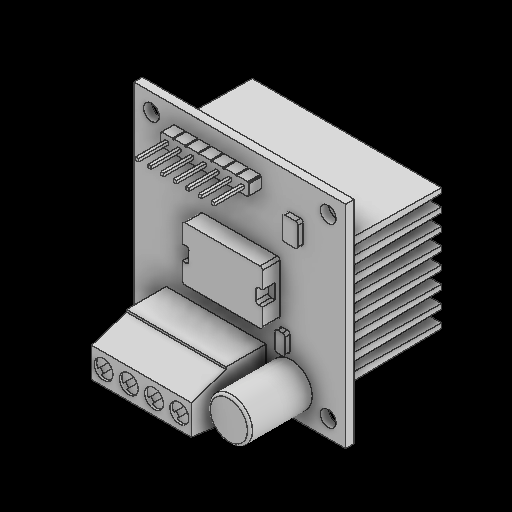
# Autodesk Inventor part: IBTMiniOriginal
Saved by Autodesk Inventor 2025.2 (Build 292293000, 293)
## iProperties
Created: 2023-12-09
Part Number: IBTMiniOriginal
Material: Generic
Document SubType Name: Modeling
Designer: valer
Density: 1 g/cm^3
Appearance: Default
Author: valer
Autodesk Inventor part; units mm, degrees
ref_plane "YZ Plane" through (0, 0, 0) normal (1, 0, 0) x (0, 1, 0)
ref_plane "XZ Plane" through (0, 0, 0) normal (0, 1, 0) x (-1, 0, 0)
ref_plane "XY Plane" through (0, 0, 0) normal (0, 0, 1) x (1, 0, 0)
sketch "Sketch1" plane through (0, 0, 0) normal (0, 0, 1) x (1, 0, 0)
  line L0 (-21.25, 21.25) -> (21.25, 21.25)
  line L1 (21.25, 21.25) -> (21.25, -21.25)
  line L2 (21.25, -21.25) -> (-21.25, -21.25)
  line L3 (-21.25, -21.25) -> (-21.25, 21.25)
  line L4 (-29.75, 0) -> (29.75, 0) construction
  line L5 (0, -29.75) -> (0, 29.75) construction
  point P0 (0, 0)
  point P1 (0, 21.25)
  point P2 (-21.25, 0)
  dimension "d0" = 42.5
  constraints: 8 end point, 2 midpoint, 2 parallel, 2 perpendicular, 2 point on line, 1 horizontal
  measures "d0" distance of L0.start L0.end
extrude "Extrusion1" add sketch "Sketch1" along normal blind 1.7
sketch "Sketch2" plane through (0, 0, 1.7) normal (0, 0, 1) x (1, 0, 0)
  circle A0 centre (-17.75, 17.75) radius 3.5 construction
  line L0 (21.25, 21.25) -> (-21.25, 21.25) construction
  line L1 (-21.25, 21.25) -> (-21.25, -21.25) construction
  circle A1 centre (-17.75, 17.75) radius 1.6
  line L2 (-17.75, 19.35) -> (-17.75, 21.25) construction
  line L3 (-19.35, 17.75) -> (-21.25, 17.75) construction
  line L4 (-29.75, 0) -> (29.75, 0) construction
  line L5 (0, -29.75) -> (0, 29.75) construction
  circle A2 centre (17.75, 17.75) radius 1.6
  circle A3 centre (-17.75, -17.75) radius 1.6
  circle A4 centre (17.75, -17.75) radius 1.6
  point P0 (0, 0)
  dimension "d3" = 1.9
  dimension "d4" = 3.2
  constraints: 5 centre point, 4 end point, 4 point on circle, 3 perpendicular, 3 symmetric about line, 2 point on line, 2 tangent, 1 coincident, 3 other
  measures "d3" distance of L2.start L2.end
  measures "d4" diameter of A1
extrude "Extrusion2" cut sketch "Sketch2" against normal blind 1.7
sketch "Sketch3" plane through (0, 0, 1.7) normal (0, 0, 1) x (1, 0, 0)
  line L0 (-21.25, 21.25) -> (-21.25, -21.25) construction
  line L1 (-21.25, 0) -> (21.25, 0) construction
  line L2 (21.25, -21.25) -> (21.25, 21.25) construction
  line L3 (-8.05, 5.4) -> (8.05, 5.4)
  line L4 (8.05, 5.4) -> (8.05, -5.4)
  line L5 (8.05, -5.4) -> (-8.05, -5.4)
  line L6 (-8.05, -5.4) -> (-8.05, 5.4)
  line L7 (0, -29.75) -> (0, 29.75) construction
  point P0 (0, 0)
  point P1 (-8.05, 0)
  point P2 (0, 5.4)
  dimension "d7" = 16.1
  dimension "d8" = 10.8
  constraints: 10 end point, 4 midpoint, 2 parallel, 2 point on line, 1 horizontal, 1 perpendicular
  measures "d7" distance of L3.start L3.end
  measures "d8" distance of L3.end L4.end
extrude "Extrusion3" add sketch "Sketch3" along normal blind 3.5
sketch "Sketch4" plane through (0, 0, 5.2) normal (0, 0, 1) x (1, 0, 0)
  line L0 (-8.05, -5.4) -> (8.05, -5.4) projected
  line L1 (8.05, -5.4) -> (8.05, 5.4) projected
  line L2 (8.05, 5.4) -> (-8.05, 5.4) projected
  line L3 (-8.05, 5.4) -> (-8.05, -5.4) projected
  line L4 (6.75, 1.5) -> (8.05, 1.5)
  line L5 (8.05, 1.5) -> (8.05, -1.5)
  line L6 (8.05, -1.5) -> (6.75, -1.5)
  line L7 (6.75, -1.5) -> (6.75, 1.5)
  line L8 (0, -29.75) -> (0, 29.75) construction
  line L9 (-6.75, 1.5) -> (-8.05, 1.5)
  line L10 (-8.05, 1.5) -> (-8.05, -1.5)
  line L11 (-8.05, -1.5) -> (-6.75, -1.5)
  line L12 (-6.75, -1.5) -> (-6.75, 1.5)
  point P0 (0, 0)
  point P1 (8.05, 0)
  dimension "d11" = 3
  dimension "d12" = 1.3
  constraints: 16 end point, 4 symmetric about line, 2 midpoint, 2 parallel, 1 horizontal, 1 perpendicular
  measures "d11" distance of L6.end L4.start
  measures "d12" distance of L5.end L6.end
extrude "Extrusion4" cut sketch "Sketch4" against normal blind 2.5 contours L3 L9 L12 L11 | L6 L7 L4 L1
fillet "Fillet1" radius 0.5 4 edges at (6.75, 1.5, 3.95) (6.75, -1.5, 3.95) (-6.75, 1.5, 3.95) (-6.75, -1.5, 3.95)
sketch "Sketch5" plane through (0, 0, 1.7) normal (0, 0, 1) x (1, 0, 0)
  circle A0 centre (10.3, -15.5) radius 4.25
  line L0 (-15.45, -11.25) -> (4.35, -11.25)
  line L1 (4.35, -11.25) -> (4.35, -19.75)
  line L2 (4.35, -19.75) -> (-15.45, -19.75)
  line L3 (-15.45, -19.75) -> (-15.45, -11.25)
  line L4 (-13.45, 17.85) -> (4.35, 17.85)
  line L5 (4.35, 17.85) -> (4.35, 15.25)
  line L6 (4.35, 15.25) -> (-13.45, 15.25)
  line L7 (-13.45, 15.25) -> (-13.45, 17.85)
  line L8 (21.25, 21.25) -> (-21.25, 21.25) projected
  line L9 (-21.25, 21.25) -> (-21.25, -21.25) projected
  line L10 (-15.45, -15.5) -> (14.55, -15.5) construction
  line L11 (4.35, -11.25) -> (10.3, -11.25) construction
  line L12 (-21.25, -21.25) -> (21.25, -21.25) construction
  line L13 (21.25, -21.25) -> (21.25, 21.25) projected
  point P0 (0, 0)
  point P1 (-13.45, 16.55)
  dimension "d16" = 17.8
  dimension "d17" = 2.6
  dimension "d18" = 7.8
  dimension "d19" = 3.4
  dimension "d20" = 30
  dimension "d21" = 8.5
  dimension "d22" = 1.5
  dimension "d23" = 6.7
  constraints: 20 end point, 5 parallel, 2 horizontal, 2 midpoint, 2 perpendicular, 2 point on circle, 2 point on line, 1 centre point, 1 collinear, 1 tangent
  measures "d16" distance of L5.end L6.end
  measures "d17" distance of L4.end L5.end
  measures "d18" distance from line of L9 point (-13.45, 16.55)
  measures "d19" distance between parallel lines of L8 L4
  measures "d20" distance of L10.end L10.start
  measures "d21" distance of L2.end L0.start
  measures "d22" distance between parallel lines of L12 L2
  measures "d23" distance from line of L13 L10.end
extrude "Extrusion5" add sketch "Sketch5" along normal blind 12.5 contours A0
extrude "Extrusion6" add sketch "Sketch5" along normal blind 2.5 contours L4 L5 L6 L7
fillet "Fillet2" radius 0.5 1 edges at (6.05, -15.5, 14.2)
sketch "Sketch8" plane through (0, 0, 1.7) normal (0, 0, 1) x (1, 0, 0)
  line L0 (9.525, 9.525) -> (12.7, 9.525)
  line L1 (12.7, 9.525) -> (12.7, 14.2875)
  line L2 (12.7, 14.2875) -> (9.525, 14.2875)
  line L3 (9.525, 14.2875) -> (9.525, 9.525)
  point P0 (0, 0)
  dimension "d60" = 3.175
  dimension "d61" = 4.7625
  dimension "d62" = 12.7
  dimension "d63" = 14.2875
  constraints: 8 end point, 2 parallel, 1 horizontal, 1 perpendicular
  measures "d60" distance between parallel lines of L1 L3
  measures "d61" distance between parallel lines of L0 L2
  measures "d62" distance from line of point (0, 0) L1
  measures "d63" distance from line of point (0, 0) L2
extrude "Extrusion9" add sketch "Sketch8" along normal blind 1
sketch "Sketch9" plane through (0, 0, 0) normal (0, 0, -1) x (-1, 0, 0)
  line L0 (19, -12.55) -> (-19, -12.55)
  line L1 (-19, -12.55) -> (-19, 12.55)
  line L2 (-19, 12.55) -> (19, 12.55)
  line L3 (19, 12.55) -> (19, -12.55)
  line L4 (29.75, 0) -> (-29.75, 0) projected
  line L5 (0, -29.75) -> (0, 29.75) projected
  point P0 (0, 0)
  point P1 (0, -12.55)
  point P2 (19, 0)
  dimension "d66" = 25.1
  dimension "d67" = 38
  constraints: 8 end point, 2 midpoint, 2 parallel, 2 point on line, 1 horizontal, 1 perpendicular
  measures "d66" distance of L0.end L1.end
  measures "d67" distance of L0.start L0.end
extrude "Extrusion10" add sketch "Sketch9" along normal blind 19.8
sketch "Sketch11" plane through (0, 0, 1.7) normal (0, 0, 1) x (1, 0, 0)
  line L0 (8.05, -6.48) -> (10.05, -6.48)
  line L1 (10.05, -6.48) -> (10.05, -10.48)
  line L2 (10.05, -10.48) -> (8.05, -10.48)
  line L3 (8.05, -10.48) -> (8.05, -6.48)
  line L4 (21.25, -21.25) -> (21.25, 21.25) projected
  line L5 (-21.25, -21.25) -> (21.25, -21.25) projected
  point P0 (0, 0)
  point P1 (10.05, -8.48)
  dimension "d79" = 2
  dimension "d80" = 4
  dimension "d81" = 11.2
  dimension "d82" = 10.77
  constraints: 8 end point, 2 parallel, 1 horizontal, 1 midpoint, 1 perpendicular
  measures "d79" distance of L0.start L0.end
  measures "d80" distance of L0.end L1.end
  measures "d81" distance from line of L4 point (10.05, -8.48)
  measures "d82" distance between parallel lines of L5 L2
extrude "LedFeature" add sketch "Sketch11" along normal blind 1
sketch "Sketch12" plane through (19, -12.55, 0) normal (1, 0, 0) x (0, 0, -1)
  line L0 (0, -8.7) -> (0, 33.8) projected
  line L1 (0, 0) -> (19.8, 0) projected
  line L2 (2, 0) -> (2, 25.1)
  line L3 (0, 25.1) -> (19.8, 25.1) projected
  line L4 (2, 0) -> (19.8, 0.3)
  line L5 (19.8, 25.1) -> (19.8, 0) projected
  line L6 (19.8, 0.3) -> (19.8, 1.3)
  line L7 (19.8, 1.3) -> (2, 1.6)
  line L8 (19.8, 0.8) -> (2, 0.8) construction
  line L9 (2, 12.55) -> (19.8, 12.55) construction
  line L10 (2, 25.1) -> (19.8, 24.8)
  line L11 (19.8, 24.8) -> (19.8, 23.8)
  line L12 (19.8, 23.8) -> (2, 23.5)
  line L13 (2, 3.3571) -> (19.8, 3.6571)
  line L14 (19.8, 3.6571) -> (19.8, 4.6571)
  line L15 (19.8, 4.6571) -> (2, 4.9571)
  line L16 (19.8, 4.1571) -> (2, 4.1571) construction
  line L17 (2, 6.7143) -> (19.8, 7.0143)
  line L18 (19.8, 7.0143) -> (19.8, 8.0143)
  line L19 (19.8, 8.0143) -> (2, 8.3143)
  line L20 (19.8, 7.5143) -> (2, 7.5143) construction
  line L21 (2, 10.0714) -> (19.8, 10.3714)
  line L22 (19.8, 10.3714) -> (19.8, 11.3714)
  line L23 (19.8, 11.3714) -> (2, 11.6714)
  line L24 (19.8, 10.8714) -> (2, 10.8714) construction
  line L25 (2, 21.7429) -> (19.8, 21.4429)
  line L26 (19.8, 20.4429) -> (2, 20.1429)
  line L27 (2, 18.3857) -> (19.8, 18.0857)
  line L28 (19.8, 17.0857) -> (2, 16.7857)
  line L29 (2, 15.0286) -> (19.8, 14.7286)
  line L30 (19.8, 13.7286) -> (2, 13.4286)
  point P0 (0, 12.55)
  point P1 (2, 23.5)
  point P2 (2, 20.1429)
  point P3 (2, 16.7857)
  point P4 (2, 13.4286)
  dimension "d85" = 2
  dimension "d86" = 1.6
  dimension "d87" = 1
  dimension "d88" = 1.7571
  dimension "d89" = 1.7571
  dimension "d90" = 1.7571
  dimension "d91" = 0.8786
  dimension "d92" = 90.966
  dimension "d93" = 90.966
  dimension "d94" = 90.966
  dimension "d95" = 90.966
  dimension "d96" = 90.966
  dimension "d97" = 90.966
  constraints: 52 end point, 15 symmetric about line, 6 equal length, 4 horizontal, 4 midpoint, 2 point on line, 1 vertical, 24 other
  measures "d86" distance of L7.end L4.start
  measures "d87" distance of L6.end L4.end
  measures "d88" distance of L13.start L7.end
  measures "d89" distance of L17.start L15.end
  measures "d90" distance of L21.start L19.end
  measures "d91" distance of L9.start L23.end
extrude "Extrusion13" cut sketch "Sketch12" against normal through all contours L4 L5 L1 | L3 L5 L10 | L2 L13 L5 L7 | L12 L5 L25 L2 | L2 L17 L5 L15 | L26 L5 L27 L2 | L2 L21 L5 L19 | L28 L5 L29 L2 | L2 L30 L5 L23
sketch "Sketch14" plane through (0, 0, 4.2) normal (0, 0, 1) x (1, 0, 0)
  line L0 (-13.45, 15.25) -> (4.35, 15.25) construction
  line L1 (4.35, 15.25) -> (4.35, 17.85) construction
  line L2 (4.35, 17.85) -> (-13.45, 17.85) construction
  line L3 (-13.45, 17.85) -> (-13.45, 15.25) construction
  line L4 (-13.45, 15.25) -> (4.35, 15.25) construction
  line L5 (1.8071, 15.25) -> (1.8071, 17.85) construction
  line L6 (-13.45, 17.85) -> (-13.45, 15.25) projected
  line L7 (4.35, 15.25) -> (1.8071, 17.85) construction
  line L8 (3.3786, 16.85) -> (2.7786, 16.85)
  line L9 (2.7786, 16.85) -> (2.7786, 16.25)
  line L10 (2.7786, 16.25) -> (3.3786, 16.25)
  line L11 (3.3786, 16.25) -> (3.3786, 16.85)
  line L12 (3.3786, 16.85) -> (2.7786, 16.25) construction
  line L13 (2.7786, 16.85) -> (3.3786, 16.25) construction
  line L14 (0.2357, 16.25) -> (0.8357, 16.25)
  line L15 (0.8357, 16.25) -> (0.8357, 16.85)
  line L16 (0.2357, 16.85) -> (0.2357, 16.25)
  line L17 (0.8357, 16.85) -> (0.2357, 16.85)
  line L18 (-2.3071, 16.25) -> (-1.7071, 16.25)
  line L19 (-1.7071, 16.25) -> (-1.7071, 16.85)
  line L20 (-2.3071, 16.85) -> (-2.3071, 16.25)
  line L21 (-1.7071, 16.85) -> (-2.3071, 16.85)
  line L22 (-4.85, 16.25) -> (-4.25, 16.25)
  line L23 (-4.25, 16.25) -> (-4.25, 16.85)
  line L24 (-4.85, 16.85) -> (-4.85, 16.25)
  line L25 (-4.25, 16.85) -> (-4.85, 16.85)
  line L26 (-7.3929, 16.25) -> (-6.7929, 16.25)
  line L27 (-6.7929, 16.25) -> (-6.7929, 16.85)
  line L28 (-7.3929, 16.85) -> (-7.3929, 16.25)
  line L29 (-6.7929, 16.85) -> (-7.3929, 16.85)
  line L30 (-9.9357, 16.25) -> (-9.3357, 16.25)
  line L31 (-9.3357, 16.25) -> (-9.3357, 16.85)
  line L32 (-9.9357, 16.85) -> (-9.9357, 16.25)
  line L33 (-9.3357, 16.85) -> (-9.9357, 16.85)
  line L34 (-12.4786, 16.25) -> (-11.8786, 16.25)
  line L35 (-11.8786, 16.25) -> (-11.8786, 16.85)
  line L36 (-12.4786, 16.85) -> (-12.4786, 16.25)
  line L37 (-11.8786, 16.85) -> (-12.4786, 16.85)
  point P0 (0, 0)
  point P1 (-13.45, 16.55)
  point P2 (4.35, 16.55)
  point P3 (3.0786, 16.55)
  dimension "d100" = 17.8
  dimension "d101" = 2.5429
  dimension "d102" = 0.6
  dimension "d105" = 2.5429
  constraints: 64 end point, 5 midpoint, 3 perpendicular, 2 horizontal, 2 parallel, 2 point on line, 48 other
  measures "d100" distance of point (-13.45, 16.55) point (4.35, 16.55)
  measures "d101" distance between parallel lines of L5 L1
  measures "d102" distance of L8.end L9.end
  measures "d105" distance of L9.end L14.start
extrude "Extrusion14" add sketch "Sketch14" along normal blind 6
fillet "Fillet3" radius 0.5 12 edges at (8.05, 5.4, 3.45) (-8.05, 5.4, 3.45) (8.05, -5.4, 3.45) (-8.05, -5.4, 3.45) (10.05, -6.48, 2.2) (8.05, -6.48, 2.2) (10.05, -10.48, 2.2) (8.05, -10.48, 2.2) (12.7, 9.525, 2.2) (12.7, 14.2875, 2.2) (9.525, 14.2875, 2.2) (9.525, 9.525, 2.2)
sketch "Sketch15" plane through (0, 0, 1.7) normal (0, 0, 1) x (1, 0, 0)
  line L0 (-21.25, -21.25) -> (21.25, -21.25) projected
  line L1 (-14.75, -11.05) -> (5.25, -11.05)
  line L2 (5.25, -11.05) -> (5.25, -21.25)
  line L3 (5.25, -21.25) -> (-14.75, -21.25)
  line L4 (-14.75, -21.25) -> (-14.75, -11.05)
  line L5 (-21.25, 21.25) -> (-21.25, -21.25) projected
  point P0 (0, 0)
  dimension "d113" = 20
  dimension "d114" = 6.5
  dimension "d115" = 10.2
  constraints: 8 end point, 2 parallel, 1 horizontal, 1 perpendicular, 1 point on line
  measures "d113" distance of L1.start L1.end
  measures "d114" distance between parallel lines of L5 L4
  measures "d115" distance of L3.end L1.start
extrude "Extrusion15" add sketch "Sketch15" along normal blind 8
sketch "Sketch16" plane through (-14.75, -21.25, 1.7) normal (-1, 0, 0) x (0, 0, 1)
  line L0 (8, 10.2) -> (8, 0) projected
  line L1 (8, 0.5) -> (15, 1.4838)
  line L2 (15, 1.4838) -> (15, 7.4838)
  line L3 (15, 7.4838) -> (6.6404, 10.2)
  line L4 (0, 10.2) -> (8, 10.2) projected
  point P0 (-1.7, 21.25)
  point P1 (8, 9.7582)
  dimension "d118" = 0.5
  dimension "d119" = 7
  dimension "d120" = 6
  dimension "d121" = 72
  dimension "d122" = 82
  constraints: 6 end point, 2 point on line, 1 parallel
  measures "d118" distance of L0.end L1.start
  measures "d119" distance between parallel lines of L0 L2
  measures "d120" distance of L1.end L2.end
  measures "d121" angle of L0 L3
  measures "d122" angle of L0 L1
extrude "Extrusion16" add sketch "Sketch16" against normal up to surface (20 mm away) contours L3 L2 L1 L0
sketch "Sketch17" plane through (0, 0, 4.2) normal (0, 0, 1) x (1, 0, 0)
  line L0 (-13.45, 15.25) -> (4.35, 15.25) construction
  line L1 (-13.45, 17.85) -> (-13.45, 15.25) construction
  line L2 (4.35, 17.85) -> (-13.45, 17.85) construction
  line L3 (4.35, 15.25) -> (4.35, 17.85) construction
  line L4 (-9.9357, 16.85) -> (-9.9357, 16.25) construction
  line L5 (-9.9357, 16.55) -> (-11.8786, 16.55) construction
  line L6 (-11.8786, 16.25) -> (-11.8786, 16.85) construction
  line L7 (-10.7821, 17.85) -> (-11.0321, 17.85) construction
  line L8 (-11.0321, 17.85) -> (-11.0321, 15.25) construction
  line L9 (-11.0321, 15.25) -> (-10.7821, 15.25) construction
  line L10 (-10.7821, 15.25) -> (-10.7821, 17.85) construction
  line L11 (-10.7821, 17.85) -> (-11.0321, 15.25) construction
  line L12 (-11.0321, 17.85) -> (-10.7821, 15.25) construction
  line L13 (4.35, 15.5) -> (-13.45, 15.5) construction
  line L14 (4.35, 17.6) -> (-13.45, 17.6) construction
  line L15 (-9.3357, 16.25) -> (-9.3357, 16.85) construction
  line L16 (-9.3357, 16.55) -> (-7.3929, 16.55) construction
  line L17 (-7.3929, 16.25) -> (-7.3929, 16.85) construction
  line L18 (-6.7929, 16.85) -> (-6.7929, 16.25) construction
  line L19 (-6.7929, 16.55) -> (-4.85, 16.55) construction
  line L20 (-4.85, 16.85) -> (-4.85, 16.25) construction
  line L21 (-4.25, 16.25) -> (-4.25, 16.85) construction
  line L22 (-4.25, 16.55) -> (-2.3071, 16.55) construction
  line L23 (-2.3071, 16.25) -> (-2.3071, 16.85) construction
  line L24 (-1.7071, 16.85) -> (-1.7071, 16.25) construction
  line L25 (-1.7071, 16.55) -> (0.2357, 16.55) construction
  line L26 (0.2357, 16.85) -> (0.2357, 16.25) construction
  line L27 (0.8357, 16.25) -> (0.8357, 16.85) construction
  line L28 (0.8357, 16.55) -> (2.7786, 16.55) construction
  line L29 (2.7786, 16.85) -> (2.7786, 16.25) construction
  line L30 (-8.2393, 17.85) -> (-8.4893, 17.85) construction
  line L31 (-8.4893, 17.85) -> (-8.4893, 15.25) construction
  line L32 (-8.4893, 15.25) -> (-8.2393, 15.25) construction
  line L33 (-8.2393, 15.25) -> (-8.2393, 17.85) construction
  line L34 (-8.2393, 17.85) -> (-8.4893, 15.25) construction
  line L35 (-8.4893, 17.85) -> (-8.2393, 15.25) construction
  line L36 (-5.6964, 17.85) -> (-5.9464, 17.85) construction
  line L37 (-5.9464, 17.85) -> (-5.9464, 15.25) construction
  line L38 (-5.9464, 15.25) -> (-5.6964, 15.25) construction
  line L39 (-5.6964, 15.25) -> (-5.6964, 17.85) construction
  line L40 (-5.6964, 17.85) -> (-5.9464, 15.25) construction
  line L41 (-5.9464, 17.85) -> (-5.6964, 15.25) construction
  line L42 (-3.1536, 17.85) -> (-3.4036, 17.85) construction
  line L43 (-3.4036, 17.85) -> (-3.4036, 15.25) construction
  line L44 (-3.4036, 15.25) -> (-3.1536, 15.25) construction
  line L45 (-3.1536, 15.25) -> (-3.1536, 17.85) construction
  line L46 (-3.1536, 17.85) -> (-3.4036, 15.25) construction
  line L47 (-3.4036, 17.85) -> (-3.1536, 15.25) construction
  line L48 (-0.6107, 17.85) -> (-0.8607, 17.85) construction
  line L49 (-0.8607, 17.85) -> (-0.8607, 15.25) construction
  line L50 (-0.8607, 15.25) -> (-0.6107, 15.25) construction
  line L51 (-0.6107, 15.25) -> (-0.6107, 17.85) construction
  line L52 (-0.6107, 17.85) -> (-0.8607, 15.25) construction
  line L53 (-0.8607, 17.85) -> (-0.6107, 15.25) construction
  line L54 (1.9321, 17.85) -> (1.6821, 17.85) construction
  line L55 (1.6821, 17.85) -> (1.6821, 15.25) construction
  line L56 (1.6821, 15.25) -> (1.9321, 15.25) construction
  line L57 (1.9321, 15.25) -> (1.9321, 17.85) construction
  line L58 (1.9321, 17.85) -> (1.6821, 15.25) construction
  line L59 (1.6821, 17.85) -> (1.9321, 15.25) construction
  line L60 (1.9321, 15.5) -> (1.6821, 15.5)
  line L61 (1.6821, 15.5) -> (1.6821, 15.25)
  line L62 (1.6821, 15.25) -> (1.9321, 15.25)
  line L63 (1.9321, 15.25) -> (1.9321, 15.5)
  line L64 (1.9321, 17.6) -> (1.6821, 17.6)
  line L65 (1.6821, 17.6) -> (1.6821, 17.85)
  line L66 (1.6821, 17.85) -> (1.9321, 17.85)
  line L67 (1.9321, 17.85) -> (1.9321, 17.6)
  line L68 (-0.6107, 15.5) -> (-0.8607, 15.5)
  line L69 (-0.8607, 15.5) -> (-0.8607, 15.25)
  line L70 (-0.8607, 15.25) -> (-0.6107, 15.25)
  line L71 (-0.6107, 15.25) -> (-0.6107, 15.5)
  line L72 (-0.6107, 17.85) -> (-0.8607, 17.85)
  line L73 (-0.8607, 17.85) -> (-0.8607, 17.6)
  line L74 (-0.8607, 17.6) -> (-0.6107, 17.6)
  line L75 (-0.6107, 17.6) -> (-0.6107, 17.85)
  line L76 (-3.1536, 17.6) -> (-3.4036, 17.6)
  line L77 (-3.4036, 17.6) -> (-3.4036, 17.85)
  line L78 (-3.4036, 17.85) -> (-3.1536, 17.85)
  line L79 (-3.1536, 17.85) -> (-3.1536, 17.6)
  line L80 (-3.1536, 15.25) -> (-3.4036, 15.25)
  line L81 (-3.4036, 15.25) -> (-3.4036, 15.5)
  line L82 (-3.4036, 15.5) -> (-3.1536, 15.5)
  line L83 (-3.1536, 15.5) -> (-3.1536, 15.25)
  line L84 (-5.6964, 17.85) -> (-5.9464, 17.85)
  line L85 (-5.9464, 17.85) -> (-5.9464, 17.6)
  line L86 (-5.9464, 17.6) -> (-5.6964, 17.6)
  line L87 (-5.6964, 17.6) -> (-5.6964, 17.85)
  line L88 (-5.6964, 15.25) -> (-5.9464, 15.25)
  line L89 (-5.9464, 15.25) -> (-5.9464, 15.5)
  line L90 (-5.9464, 15.5) -> (-5.6964, 15.5)
  line L91 (-5.6964, 15.5) -> (-5.6964, 15.25)
  line L92 (-8.2393, 17.85) -> (-8.4893, 17.85)
  line L93 (-8.4893, 17.85) -> (-8.4893, 17.6)
  line L94 (-8.4893, 17.6) -> (-8.2393, 17.6)
  line L95 (-8.2393, 17.6) -> (-8.2393, 17.85)
  line L96 (-8.2393, 15.25) -> (-8.4893, 15.25)
  line L97 (-8.4893, 15.25) -> (-8.4893, 15.5)
  line L98 (-8.4893, 15.5) -> (-8.2393, 15.5)
  line L99 (-8.2393, 15.5) -> (-8.2393, 15.25)
  line L100 (-10.7821, 17.6) -> (-11.0321, 17.6)
  line L101 (-11.0321, 17.6) -> (-11.0321, 17.85)
  line L102 (-11.0321, 17.85) -> (-10.7821, 17.85)
  line L103 (-10.7821, 17.85) -> (-10.7821, 17.6)
  line L104 (-10.7821, 15.25) -> (-11.0321, 15.25)
  line L105 (-11.0321, 15.25) -> (-11.0321, 15.5)
  line L106 (-11.0321, 15.5) -> (-10.7821, 15.5)
  line L107 (-10.7821, 15.5) -> (-10.7821, 15.25)
  line L108 (4.35, 17.85) -> (4.1, 17.85)
  line L109 (4.1, 17.85) -> (4.1, 17.6)
  line L110 (4.1, 17.6) -> (4.35, 17.6)
  line L111 (4.35, 17.6) -> (4.35, 17.85)
  line L112 (4.35, 15.5) -> (4.1, 15.5)
  line L113 (4.1, 15.5) -> (4.1, 15.25)
  line L114 (4.1, 15.25) -> (4.35, 15.25)
  line L115 (4.35, 15.25) -> (4.35, 15.5)
  line L116 (-13.45, 17.85) -> (-13.2, 17.85)
  line L117 (-13.2, 17.85) -> (-13.2, 17.6)
  line L118 (-13.2, 17.6) -> (-13.45, 17.6)
  line L119 (-13.45, 17.6) -> (-13.45, 17.85)
  line L120 (-13.45, 15.25) -> (-13.2, 15.25)
  line L121 (-13.2, 15.25) -> (-13.2, 15.5)
  line L122 (-13.2, 15.5) -> (-13.45, 15.5)
  line L123 (-13.45, 15.5) -> (-13.45, 15.25)
  point P0 (0, 0)
  point P1 (-10.9071, 16.55)
  point P2 (-8.3643, 16.55)
  point P3 (-5.8214, 16.55)
  point P4 (-3.2786, 16.55)
  point P5 (-0.7357, 16.55)
  point P6 (1.8071, 16.55)
  dimension "d126" = 0.25
  dimension "d125" = 0.25
  dimension "d128" = 2.4179
  dimension "d129" = 0.25
  dimension "d130" = 0.25
  constraints: 212 end point, 44 parallel, 30 midpoint, 22 horizontal, 22 perpendicular, 16 point on line, 5 collinear, 2 symmetric about line, 1 vertical, 29 other
  measures "d125" distance between parallel lines of L8 L10
  measures "d128" distance between parallel lines of L1 L8
  measures "d129" distance between parallel lines of L109 L3
  measures "d130" distance between parallel lines of L1 L117
extrude "Extrusion17" cut sketch "Sketch17" against normal up to surface (2.5 mm away)
sketch "Sketch18" plane through (-14.75, -19.7662, 16.7) normal (0, 0, 1) x (1, 0, 0)
  line L0 (20, 0) -> (20, 6) construction
  line L1 (20, 3) -> (0, 3) construction
  line L2 (0, 0) -> (0, 6) construction
  circle A0 centre (17.6, 3) radius 1.9
  line L3 (15.7, 4.9) -> (19.5, 4.9) construction
  line L4 (19.5, 4.9) -> (19.5, 1.1) construction
  line L5 (19.5, 1.1) -> (15.7, 1.1) construction
  line L6 (15.7, 1.1) -> (15.7, 4.9) construction
  line L7 (15.7, 4.9) -> (19.5, 1.1) construction
  line L8 (19.5, 4.9) -> (15.7, 1.1) construction
  line L9 (0, 6) -> (20, 6) construction
  line L10 (10, 6) -> (10, 0) construction
  line L11 (0, 0) -> (20, 0) construction
  circle A1 centre (2.4, 3) radius 1.9
  circle A2 centre (12.5333, 3) radius 1.9
  circle A3 centre (7.4667, 3) radius 1.9
  point P0 (14.75, 19.7662)
  dimension "d133" = 3.8
  dimension "d134" = 0.5
  dimension "d135" = 5.0667
  dimension "d136" = 5.0667
  dimension "d137" = 5.0667
  constraints: 16 end point, 6 midpoint, 4 centre point, 3 point on line, 2 equal radius, 2 parallel, 2 tangent, 1 horizontal, 1 perpendicular, 1 symmetric about line, 1 other
  measures "d133" diameter of A0
  measures "d134" distance between parallel lines of L0 L4
  measures "d135" distance of A2.centre A0.centre
  measures "d136" distance of A3.centre A2.centre
  measures "d137" distance of A1.centre A3.centre
extrude "Extrusion18" cut sketch "Sketch18" against normal blind 0.5
sketch "Sketch19" plane through (2.85, -16.7662, 16.2) normal (0, 0, 1) x (1, 0, 0)
  circle A0 centre (0, 0) radius 1.9 projected
  line L0 (1.3435, 1.3435) -> (-1.3435, -1.3435) construction
  line L1 (1.6497, 0.9426) -> (-0.9426, -1.6497)
  line L2 (-1.6497, -0.9426) -> (0.9426, 1.6497)
  line L3 (-32.6, 16.7662) -> (26.9, 16.7662) construction
  circle A1 centre (-5.0667, 0) radius 1.9 projected
  circle A2 centre (-10.1333, 0) radius 1.9 projected
  circle A3 centre (-15.2, 0) radius 1.9 projected
  line L4 (-3.417, 0.9426) -> (-6.0093, -1.6497)
  line L5 (-6.7164, -0.9426) -> (-4.1241, 1.6497)
  line L6 (-8.4836, 0.9426) -> (-11.0759, -1.6497)
  line L7 (-11.783, -0.9426) -> (-9.1907, 1.6497)
  line L8 (-13.5503, 0.9426) -> (-16.1426, -1.6497)
  line L9 (-16.8497, -0.9426) -> (-14.2574, 1.6497)
  point P0 (-2.85, 16.7662)
  point P1 (-14.2574, 1.6497)
  point P2 (-16.8497, -0.9426)
  point P3 (-16.1426, -1.6497)
  point P4 (-9.1907, 1.6497)
  point P5 (-11.783, -0.9426)
  point P6 (-11.0759, -1.6497)
  point P7 (-4.1241, 1.6497)
  point P8 (-6.7164, -0.9426)
  point P9 (-6.0093, -1.6497)
  dimension "d140" = 0.5
  dimension "d141" = 0.5
  dimension "d142" = 45
  dimension "d143" = 5.0667
  dimension "d146" = 5.0667
  constraints: 18 end point, 6 point on circle, 2 parallel, 1 coincident, 1 horizontal, 1 midpoint, 18 other
  measures "d140" distance between parallel lines of L0 L1
  measures "d141" distance between parallel lines of L2 L0
  measures "d142" angle of L3 L0
  measures "d143" distance of A1.centre A0.centre
  measures "d146" distance of L1.start L4.start
extrude "Extrusion19" cut sketch "Sketch19" against normal blind 0.5 contours L1 A0 L2 | L4 A1 L5 | L6 A2 L7 | L8 A3 L9
fillet "Fillet4" radius 0.5 1 edges at (-4.75, -21.25, 9.7)
sketch "Sketch20" plane through (0, 0, 1.7) normal (0, 0, 1) x (1, 0, 0)
  line L0 (-14.75, -21.25) -> (-14.75, -11.05) projected
  line L1 (-14.75, -13.05) -> (-15, -13.05)
  line L2 (-15, -13.05) -> (-15, -14.05)
  line L3 (-15, -14.05) -> (-14.75, -14.05)
  line L4 (-14.75, -14.05) -> (-14.75, -13.05)
  line L5 (-14.75, -20.75) -> (-15, -20.75)
  line L6 (-15, -20.75) -> (-15, -19.75)
  line L7 (-15, -19.75) -> (-14.75, -19.75)
  line L8 (-14.75, -19.75) -> (-14.75, -20.75)
  line L9 (-21.25, -21.25) -> (-14.75, -21.25) projected
  point P0 (0, 0)
  dimension "d154" = 0.5
  dimension "d155" = 1
  dimension "d156" = 2
  dimension "d157" = 0.25
  constraints: 16 end point, 4 parallel, 3 point on line, 2 horizontal, 2 perpendicular, 1 collinear
  measures "d154" distance between parallel lines of L9 L5
  measures "d155" distance of L5.end L6.end
  measures "d156" distance from line of L0.end L1
  measures "d157" distance between parallel lines of L0 L6
extrude "Extrusion20" add sketch "Sketch20" along normal up to surface (8 mm away)
sketch "Sketch21" plane through (-21.25, -21.25, 0) normal (0, -1, 0) x (1, 0, 0)
  line L0 (6.5, 16.7) -> (26.5, 16.7) construction
  line L1 (16.5, 16.7) -> (16.5, 1.7) construction
  line L2 (28.8, 1.7) -> (13.7, 1.7) construction
  line L3 (6.5, 16.7) -> (16.5, 16.7) construction
  line L4 (11.5, 16.7) -> (11.5, 1.7) construction
  line L5 (6.5, 1.7) -> (26.5, 1.7) construction
  line L6 (7.35, 7.1) -> (10.65, 7.1)
  line L7 (10.65, 7.1) -> (10.65, 3.7)
  line L8 (10.65, 3.7) -> (7.35, 3.7)
  line L9 (7.35, 3.7) -> (7.35, 7.1)
  line L10 (6.5, 9.2) -> (26.5, 9.2) construction
  line L11 (11.5, 9.2) -> (6.5, 9.2) construction
  line L12 (9, 9.2) -> (9, 1.7) construction
  line L13 (6.5, 1.7) -> (6.5, 9.2) projected
  line L14 (12.35, 7.1) -> (15.65, 7.1)
  line L15 (12.35, 3.7) -> (12.35, 7.1)
  line L16 (15.65, 7.1) -> (15.65, 3.7)
  line L17 (15.65, 3.7) -> (12.35, 3.7)
  line L18 (17.35, 7.1) -> (20.65, 7.1)
  line L19 (17.35, 3.7) -> (17.35, 7.1)
  line L20 (20.65, 7.1) -> (20.65, 3.7)
  line L21 (20.65, 3.7) -> (17.35, 3.7)
  line L22 (22.35, 7.1) -> (25.65, 7.1)
  line L23 (22.35, 3.7) -> (22.35, 7.1)
  line L24 (25.65, 7.1) -> (25.65, 3.7)
  line L25 (25.65, 3.7) -> (22.35, 3.7)
  point P0 (21.25, 0)
  point P1 (9, 7.1)
  point P2 (14, 7.1)
  point P3 (19, 7.1)
  point P4 (24, 7.1)
  dimension "d160" = 3.4
  dimension "d161" = 2
  dimension "d162" = 3.3
  dimension "d163" = 5
  dimension "d166" = 5
  constraints: 42 end point, 5 midpoint, 5 point on line, 2 collinear, 2 horizontal, 2 parallel, 2 perpendicular, 2 vertical, 27 other
  measures "d160" distance between parallel lines of L8 L6
  measures "d161" distance between parallel lines of L5 L8
  measures "d162" distance of L7.end L8.end
  measures "d163" distance between parallel lines of L4 L13
  measures "d166" distance of L6.start L14.start
extrude "Extrusion21" cut sketch "Sketch21" against normal blind 3
chamfer "Chamfer1" distance 0.25 angle 45 8 edges at (-12.25, -21.25, 3.7) (-7.25, -21.25, 3.7) (-2.25, -21.25, 3.7) (2.75, -21.25, 3.7) (2.75, -21.25, 7.1) (-2.25, -21.25, 7.1) (-7.25, -21.25, 7.1) (-12.25, -21.25, 7.1)
chamfer "Chamfer2" distance 0.25 angle 45 8 edges at (-10.6, -21.25, 5.4) (-13.9, -21.25, 5.4) (-8.9, -21.25, 5.4) (-5.6, -21.25, 5.4) (-3.9, -21.25, 5.4) (-0.6, -21.25, 5.4) (1.1, -21.25, 5.4) (4.4, -21.25, 5.4)
equation "\"d89\" = d88"
equation "\"d90\" = d88"
equation "\"d91\" = 0.5 * d88"
equation "\"d93\" = d92"
equation "\"d95\" = d92"
equation "\"d96\" = d92"
equation "\"d97\" = d92"
equation "\"d101\" = 0.142857 * d100"
equation "\"d105\" = d101"
equation "\"d136\" = d135"
equation "\"d137\" = d135"
equation "\"d141\" = d140"
equation "\"d146\" = d143"
body "Solid1"
